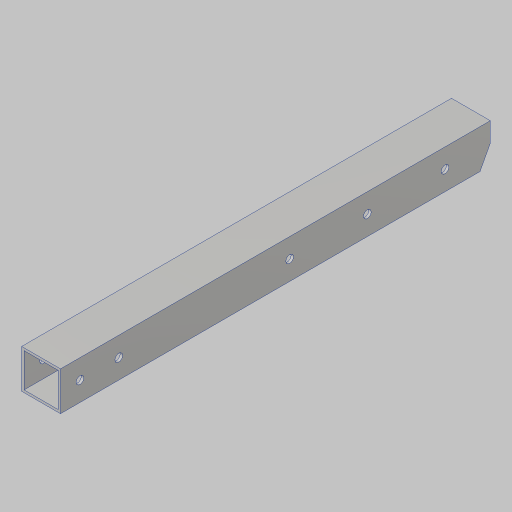
# Autodesk Inventor part: CL4-007
Saved by Autodesk Inventor 2023.5 (Build 275446000, 446)
## iProperties
RuleStatus: InUse
Created: 2025-02-03
Part Number: CL4-007
Material: Aluminum 6061
Document SubType Name: Modeling
Designer: brand
Mass: 304.185 g
Surface Area: 718.547 cm^2
Volume: 112.661 cm^3
Density: 2.7 g/cm^3
Appearance: Aluminum - Flat
AfterDocNew0: SHOW
AfterDocOpen0: SHOW
Author: brand
Autodesk Inventor part; units mm, degrees
ref_plane "YZ Plane" through (0, 0, 0) normal (1, 0, 0) x (0, 1, 0)
ref_plane "XZ Plane" through (0, 0, 0) normal (0, 1, 0) x (-1, 0, 0)
ref_plane "XY Plane" through (0, 0, 0) normal (0, 0, 1) x (1, 0, 0)
sketch "Sketch1" plane through (0, 0, 0) normal (0, 0, 1) x (1, 0, 0)
  line L0 (-12.7, -12.7) -> (12.7, -12.7)
  line L1 (12.7, -12.7) -> (12.7, 12.7)
  line L2 (12.7, 12.7) -> (-12.7, 12.7)
  line L3 (-12.7, 12.7) -> (-12.7, -12.7)
  line L4 (-12.7, -12.7) -> (12.7, 12.7) construction
  line L5 (12.7, -12.7) -> (-12.7, 12.7) construction
  line L6 (-11.1125, 11.1125) -> (11.1125, 11.1125)
  line L7 (11.1125, 11.1125) -> (11.1125, -11.1125)
  line L8 (11.1125, -11.1125) -> (-11.1125, -11.1125)
  line L9 (-11.1125, -11.1125) -> (-11.1125, 11.1125)
  point P0 (0, 0)
  dimension "width" = 25.4
  dimension "height" = 25.4
  dimension "thickness" = 1.5875
  constraints: 20 end point, 4 parallel, 2 midpoint, 2 perpendicular, 1 horizontal, 3 other
  measures "width" distance of L2.end L1.end
  measures "height" distance of L1.end L0.end
  measures "thickness" distance between parallel lines of L2 L6
extrude "Extrusion1" add sketch "Sketch1" along normal mid plane 281.1138
sketch "Sketch2" plane through (12.7, -12.7, 140.5569) normal (1, 0, 0) x (0, 0, -1)
  line L0 (281.1138, 25.4) -> (281.1138, 0) construction
  line L1 (281.1138, 0) -> (0, 0) construction
  line L2 (0, 0) -> (0, 25.4) construction
  line L3 (0, 25.4) -> (281.1138, 25.4) construction
  point P0 (140.5569, 12.7)
  point P1 (12.7, 12.7)
  point P2 (38.1, 12.7)
  point P3 (0, 12.7)
  dimension "d5" = 25.4
  dimension "d6" = 12.7
  constraints: 2 horizontal alignment, 1 midpoint
  measures "d5" distance of point (38.1, 12.7) point (12.7, 12.7)
  measures "d6" distance from line of L2 point (12.7, 12.7)
hole "Hole1" at (12.7, 0, 127.8569) at (12.7, 0, 102.4569) direction (-1, 0, 0) diameter 5.1054 end through all clearance for "Flat Head Machine Screw (82)" size "#10" standard "Ansi Unified Screw Threads"
sketch "Sketch3" plane through (12.7, -12.7, 140.5569) normal (1, 0, 0) x (0, 0, -1)
  circle A0 centre (12.7, 12.7) radius 2.5527 construction
  circle A1 centre (38.1, 12.7) radius 2.5527 construction
  line L0 (281.1138, 25.4) -> (0, 25.4) construction
  line L1 (0, 0) -> (0, 25.4) construction
  line L2 (281.1138, 0) -> (0, 0) construction
  line L3 (281.1138, 25.4) -> (281.1138, 0) construction
  line L4 (281.1138, 25.4) -> (0, 25.4) construction
  line L5 (281.1138, 25.4) -> (281.1138, 0) construction
  line L6 (274.3611, 0) -> (281.1138, 0)
  line L7 (281.1138, 0) -> (281.1138, 12.7)
  line L8 (281.1138, 12.7) -> (274.3611, 0)
  point P0 (140.5569, 12.7)
  dimension "d14" = 28
  constraints: 6 end point, 1 horizontal, 1 midpoint, 1 perpendicular, 1 point on line
  measures "d14" angle of L3 L8
extrude "Extrusion2" cut sketch "Sketch3" against normal through all
sketch "Sketch4" plane through (-12.7, -12.7, 140.5569) normal (-1, 0, 0) x (0, 0, 1)
  line L0 (-281.1138, 12.7) -> (-281.1138, 25.4) construction
  line L1 (-281.1138, 25.4) -> (0, 25.4) construction
  point P0 (-140.5569, 12.7)
  point P1 (-251.4637, 12.6978)
  point P2 (-200.6637, 12.6978)
  point P3 (-149.8637, 12.6978)
  point P4 (-281.1138, 19.05)
  dimension "d19" = 50.8
  dimension "d20" = 50.8
  dimension "d21" = 29.6501
  dimension "d22" = 12.7022
  constraints: 2 horizontal alignment, 1 midpoint
  measures "d19" distance of point (-200.664, 12.698) point (-251.464, 12.698)
  measures "d20" distance of point (-149.864, 12.698) point (-200.664, 12.698)
  measures "d21" horizontal distance of point (-281.114, 19.05) point (-251.464, 12.698)
  measures "d22" distance from line of L1 point (-251.464, 12.698)
hole "Hole2" at (-12.7, -0.0022, -110.9068) at (-12.7, -0.0022, -60.1068) at (-12.7, -0.0022, -9.3068) direction (1, 0, 0) diameter 5.1054 end through all clearance for "Flat Head Machine Screw (82)" size "#10" standard "Ansi Unified Screw Threads"
equation "\"d20\" = d19"
body "Solid1"
